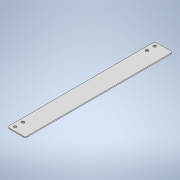
# Autodesk Inventor part: holder_ramp
Saved by Autodesk Inventor 2022 (Build 260153000, 153)
## iProperties
Created: 2021-12-26
Part Number: holder_ramp
Material: Generic
Document SubType Name: Modeling
Designer: Alex
Density: 1 g/cm^3
Appearance: Default
Author: Alex
Autodesk Inventor part; units mm, degrees
ref_plane "YZ Plane" through (0, 0, 0) normal (1, 0, 0) x (0, 1, 0)
ref_plane "XZ Plane" through (0, 0, 0) normal (0, 1, 0) x (-1, 0, 0)
ref_plane "XY Plane" through (0, 0, 0) normal (0, 0, 1) x (1, 0, 0)
sketch "Sketch1" plane through (0, 0, 0) normal (0, 1, 0) x (-1, 0, 0)
  line L0 (-3.175, 0) -> (-26.035, 0)
  line L1 (-29.21, -3.175) -> (-29.21, -238.125)
  line L2 (-26.035, -241.3) -> (-3.175, -241.3)
  line L3 (0, -238.125) -> (0, -3.175)
  circle A0 centre (-6.35, -6.35) radius 2.2225
  circle A1 centre (-6.35, -19.05) radius 2.2225
  circle A2 centre (-6.35, -234.95) radius 2.2225
  circle A3 centre (-6.35, -222.25) radius 2.2225
  arc A4 (0, -3.175) -> (-3.175, 0) centre (-3.175, -3.175) ccw
  arc A5 (-26.035, 0) -> (-29.21, -3.175) centre (-26.035, -3.175) ccw
  arc A6 (-3.175, -241.3) -> (0, -238.125) centre (-3.175, -238.125) ccw
  arc A7 (-29.21, -238.125) -> (-26.035, -241.3) centre (-26.035, -238.125) ccw
  point P0 (0, 0)
  point P1 (-29.21, -241.3)
  point P2 (-29.21, 0)
  point P3 (0, -241.3)
  dimension "d0" = 29.21
  dimension "d1" = 241.3
  dimension "d2" = 4.445
  dimension "d3" = 4.445
  dimension "d4" = 4.445
  dimension "d5" = 4.445
  dimension "d6" = 3.175
  constraints: 8 centre point, 8 end point, 8 point on circle, 8 point on line, 8 tangent, 3 equal radius, 2 parallel, 1 horizontal, 1 perpendicular
  measures "d0" distance of point (0, -241.3) point (-29.21, -241.3)
  measures "d1" distance of point (-29.21, -241.3) point (-29.21, 0)
  measures "d2" diameter of A0
  measures "d3" diameter of A1
  measures "d4" diameter of A2
  measures "d5" diameter of A3
  measures "d6" radius of A4
extrude "Extrusion1" add sketch "Sketch1" along normal blind 1.778
body "Solid1"
